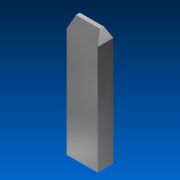
# Autodesk Inventor part: Soanar Power Module Pin A
Saved by Autodesk Inventor 2016 (Build 200138000, 138)
## iProperties
Created: 2013-08-06
Project: Power Entry Module - Soanar PP4003
Material: Nickel-Copper Alloy 400
Description: Soanar Power Module Pin A
Document SubType Name: Modeling
Designer: sdarley
Density: 8.83 g/cm^3
Appearance: Chrome - Polished
Title: Soanar Power Module Pin A
Author: sdarley
Revision Number: 1
Autodesk Inventor part; units mm, degrees
ref_plane "YZ Plane" through (0, 0, 0) normal (1, 0, 0) x (0, 1, 0)
ref_plane "XZ Plane" through (0, 0, 0) normal (0, 1, 0) x (-1, 0, 0)
ref_plane "XY Plane" through (0, 0, 0) normal (0, 0, 1) x (1, 0, 0)
sketch "Sketch1" plane through (0, 0, 0) normal (0, 1, 0) x (-1, 0, 0)
  line L0 (-2, 0) -> (2, 0)
  line L1 (2, 0) -> (2, 15.35)
  line L2 (2, 15.35) -> (-2, 15.35)
  line L3 (-2, 15.35) -> (-2, 0)
  point P0 (0, 0)
  point P1 (0, 0)
  dimension "d0" = 4
  dimension "d1" = 15.35
  constraints: 8 end point, 2 parallel, 1 coincident, 1 horizontal, 1 midpoint, 1 perpendicular
  measures "d0" distance between parallel lines of L1 L3
  measures "d1" distance between parallel lines of L0 L2
extrude "Extrusion1" add sketch "Sketch1" along normal mid plane 2
chamfer "Chamfer1" distance 1.4 distance2 0.45 1 edges at (-2, 0, 15.35) measured on face at (-2, 0.3333, 10.2333)
chamfer "Chamfer2" distance 1.4 distance2 0.45 1 edges at (2, 0, 15.35) measured on face at (2, -0.3333, 10.2333)
chamfer "Chamfer3" distance 1.4 distance2 0.75 1 edges at (0, 1, 15.35) measured on face at (0.6667, 1, 9.3)
chamfer "Chamfer4" distance 1.4 distance2 0.75 1 edges at (0, -1, 15.35) measured on face at (0.6667, -1, 9.3)
body "Solid1"
